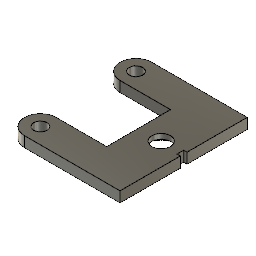
Potentiometer Bracket (Autodesk Fusion 360 design; units mm, degrees)
Autodesk Fusion 360 part; units mm, degrees
note: some values were not read from the file. Set by a fixed rule: which sketch regions a step uses.
sketch "Sketch2" plane through (0, 0, 0) normal (0, 0, 1) x (1, 0, 0)
  circle A0 centre (8.5, 12) radius 3.5
  line L0 (-25, 24) -> (-25, 36)
  line L1 (0, 0) -> (0, 24)
  line L2 (-25, 24) -> (0, 24)
  line L3 (-25, 36) -> (17, 36)
  circle A1 centre (-19, 30) radius 2.5
  circle A2 centre (8.5, 12) radius 6
  line L4 (18.25, 10.75) -> (15.75, 10.75)
  line L5 (15.75, 10.75) -> (15.75, 13.25)
  line L6 (15.75, 13.25) -> (18.25, 13.25)
  line L7 (18.25, 13.25) -> (18.25, 10.75)
  line L8 (18.25, 10.75) -> (15.75, 13.25) construction
  line L9 (15.75, 10.75) -> (18.25, 13.25) construction
  line L10 (0, 0) -> (-25, 0)
  line L11 (-25, 0) -> (-25, -12)
  line L12 (-25, -12) -> (17, -12)
  line L13 (17, -12) -> (17, 36)
  line L14 (8.5, 12) -> (17, 12) construction
  circle A3 centre (-19, -6) radius 2.5
  point P0 (17, 12)
  dimension "d16" = 7
  dimension "d20" = 12
  dimension "d21" = 25
  dimension "d22" = 12
  dimension "d23" = 5
  dimension "d25" = 12
  dimension "d30" = 2.5
  dimension "d31" = 2.5
  dimension "d34" = 6
  dimension "d35" = 6
  dimension "d36" = 12
  dimension "d37" = 25
  dimension "d38" = 17
  dimension "d39" = 8.5
  dimension "d40" = 5
  dimension "d41" = 6
  dimension "d42" = 6
  constraint coincident L1.start L10.start
  constraint perpendicular L1 L2
  constraint perpendicular L0 L2
  constraint perpendicular L0 L3
  constraint horizontal L4
  constraint perpendicular L4 L5
  constraint parallel L4 L6
  constraint parallel L5 L7
  constraint coincident L8 P0
  constraint coincident L9 P0
  constraint perpendicular L1 L10
  constraint perpendicular L10 L11
  constraint perpendicular L11 L12
  constraint perpendicular L3 L13
  constraint coincident A0.centre A2.centre
  constraint coincident L13 P0
  constraint perpendicular L13 L14
  constraint coincident P0 L14.end
  measures "d16" diameter of A0
  measures "d20" distance of L0.start L0.end
  measures "d21" distance of L0.start L1.end
  measures "d22" distance of A0.centre L2
  measures "d23" diameter of A1
  measures "d25" diameter of A2
  measures "d30" distance of L5.end L6.end
  measures "d31" distance of L4.end L5.end
  measures "d34" distance of L2 A1.centre
  measures "d35" distance of L0 A1.centre
  measures "d36" distance of L10.end L11.end
  measures "d37" distance of L1.start L10.end
  measures "d38" distance of L1.start L13
  measures "d39" distance of A0.centre L1
  measures "d40" diameter of A3
  measures "d41" distance of L11 A3.centre
  measures "d42" distance of L12 A3.centre
extrude "Extrude3" add sketch "Sketch2" along normal blind 4 contours L0 L1 L2 L3 L4 L5 L6 L10 L11 L12 L13 | L4 L5 L6 L13 | A2
extrude "Extrude4" cut sketch "Sketch2" along normal blind 2.1 contours A2
extrude "Extrude5" cut sketch "Sketch2" along normal blind 4 contours L4 L5 L6 L13
fillet "Fillet1" radius 6 4 edges at (-25, 24, 2) (-25, 0, 2) (-25, -12, 2) (-25, 36, 2)
named bodies: "Pot bracket"
